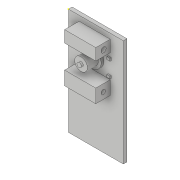
# Autodesk Inventor part: exploration.
Saved by Autodesk Inventor 2019 (Build 230136000, 136)
## iProperties
Created: 2020-02-13
Part Number: exploration.
Material: Generic
Document SubType Name: Modeling
Designer: Admin
Density: 1 g/cm^3
Appearance: Default
Author: Admin
Autodesk Inventor part; units mm, degrees
ref_plane "YZ Plane" through (0, 0, 0) normal (1, 0, 0) x (0, 1, 0)
ref_plane "XZ Plane" through (0, 0, 0) normal (0, 1, 0) x (-1, 0, 0)
ref_plane "XY Plane" through (0, 0, 0) normal (0, 0, 1) x (1, 0, 0)
sketch "Sketch1" plane through (0, 0, 0) normal (0, 0, 1) x (1, 0, 0)
  line L0 (0, 0) -> (7.6498, 0)
  line L1 (7.6498, 0) -> (7.6498, -14.8868)
  line L2 (7.6498, -14.8868) -> (0, -14.8868)
  line L3 (0, -14.8868) -> (0, 0)
  constraints: 8 end point, 2 parallel, 1 horizontal, 1 perpendicular
extrude "Extrusion1" add sketch "Sketch1" along normal blind 0.508
sketch "Sketch2" plane through (0, 0, 0.508) normal (0, 0, 1) x (1, 0, 0)
  line L0 (1.4931, -0.7177) -> (5.8329, -0.7177)
  line L1 (5.8329, -0.7177) -> (5.8329, -2.3371)
  line L2 (5.8329, -2.3371) -> (1.4931, -2.3371)
  line L3 (1.4931, -2.3371) -> (1.4931, -0.7177)
  point P0 (0, 0)
  constraints: 8 end point, 2 parallel, 1 horizontal, 1 perpendicular
extrude "Extrusion2" add sketch "Sketch2" along normal blind 2.032
sketch "Sketch3" plane through (5.8329, -2.3371, 0.508) normal (1, 0, 0) x (0, 0, -1)
  circle A0 centre (-0.9414, 0.8097) radius 0.3588
  point P0 (0.508, 2.3371)
  constraints: 1 centre point
extrude "Extrusion3" cut sketch "Sketch3" against normal blind 25.4
sketch "Sketch4" plane through (0, 0, 0.508) normal (0, 0, 1) x (1, 0, 0)
  circle A0 centre (3.6503, -3.8526) radius 1.2866
  point P0 (0, 0)
  constraints: 1 centre point
extrude "Extrusion4" add sketch "Sketch4" along normal blind 0.381
sketch "Sketch5" plane through (3.6503, -3.8526, 0.889) normal (0, 0, 1) x (1, 0, 0)
  circle A0 centre (0, 0) radius 0.8892
  point P0 (-3.6503, 3.8526)
  constraints: 1 centre point
extrude "Extrusion5" add sketch "Sketch5" along normal blind 1.524
sketch "Sketch6" plane through (3.6503, -3.8526, 2.413) normal (0, 0, 1) x (1, 0, 0)
  circle A0 centre (0, 0) radius 0.3206
  point P0 (-3.6503, 3.8526)
  constraints: 1 centre point
extrude "Extrusion6" add sketch "Sketch6" along normal blind 0.254
sketch "Sketch7" plane through (0, 0, 0.508) normal (0, 0, 1) x (1, 0, 0)
  line L0 (1.4931, -5.604) -> (5.8329, -5.604)
  line L1 (5.8329, -5.604) -> (5.8329, -7.5004)
  line L2 (5.8329, -7.5004) -> (1.4931, -7.5004)
  line L3 (1.4931, -7.5004) -> (1.4931, -5.604)
  point P0 (0, 0)
  constraints: 8 end point, 2 parallel, 1 horizontal, 1 perpendicular
extrude "Extrusion7" add sketch "Sketch7" along normal blind 2.032
sketch "Sketch8" plane through (5.8329, -7.5004, 0.508) normal (1, 0, 0) x (0, 0, -1)
  circle A0 centre (-0.993, 0.9074) radius 0.307
  point P0 (0.508, 7.5004)
  constraints: 1 centre point
extrude "Extrusion8" cut sketch "Sketch8" against normal blind 25.4 and the other way blind 12.7
sketch "Sketch9" plane through (0, 0, 0.508) normal (0, 0, 1) x (1, 0, 0)
  line L0 (1.3437, -2.8588) -> (1.7508, -2.8588)
  line L1 (1.7508, -2.8588) -> (1.7508, -3.2419)
  line L2 (1.7508, -3.2419) -> (1.3437, -3.2419)
  line L3 (1.3437, -3.2419) -> (1.3437, -2.8588)
  line L4 (5.5348, -2.8588) -> (5.9659, -2.8588)
  line L5 (5.9659, -2.8588) -> (5.9659, -3.2419)
  line L6 (5.9659, -3.2419) -> (5.5348, -3.2419)
  line L7 (5.5348, -3.2419) -> (5.5348, -2.8588)
  line L8 (1.3437, -5.0381) -> (1.7508, -5.0381)
  line L9 (1.7508, -5.0381) -> (1.7508, -5.3734)
  line L10 (1.7508, -5.3734) -> (1.3437, -5.3734)
  line L11 (1.3437, -5.3734) -> (1.3437, -5.0381)
  line L12 (5.5348, -5.0381) -> (5.9659, -5.0381)
  line L13 (5.9659, -5.0381) -> (5.9659, -5.3734)
  line L14 (5.9659, -5.3734) -> (5.5348, -5.3734)
  line L15 (5.5348, -5.3734) -> (5.5348, -5.0381)
  point P0 (0, 0)
  constraints: 32 end point, 8 parallel, 8 point on line, 4 horizontal, 4 perpendicular
extrude "Extrusion9" add sketch "Sketch9" along normal blind 0.1778
sketch "Sketch10" plane through (0, 0, 0.508) normal (0, 0, 1) x (1, 0, 0)
  point P0 (0, 0)
body "Solid1"
